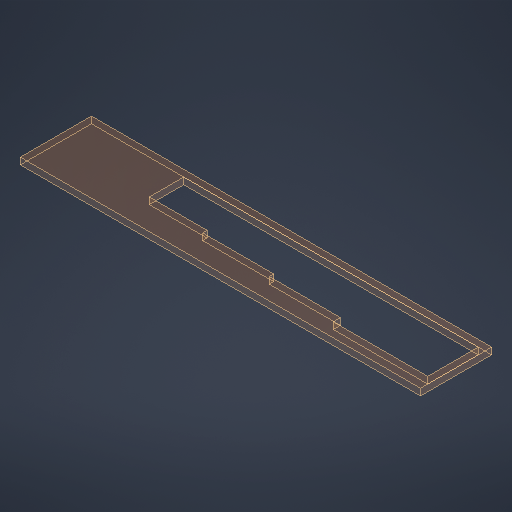
# Autodesk Inventor part: sledPlate
Saved by Autodesk Inventor 2026.1 (Build 301233020, 233B)
## iProperties
Created: 2025-11-01
Part Number: sledPlate
Material: Polycarbonate, Smoke
Document SubType Name: Modeling
Designer: Zain
Density: 1.2 g/cm^3
Appearance: Polycarbonate - Smoked
Author: Zain
Autodesk Inventor part; units mm, degrees
ref_plane "YZ Plane" through (0, 0, 0) normal (1, 0, 0) x (0, 1, 0)
ref_plane "XZ Plane" through (0, 0, 0) normal (0, 1, 0) x (-1, 0, 0)
ref_plane "XY Plane" through (0, 0, 0) normal (0, 0, 1) x (1, 0, 0)
sketch "Sketch1" plane through (0, 0, 0) normal (0, 1, 0) x (-1, 0, 0)
  line L0 (0, 0) -> (180, 0)
  line L1 (180, 0) -> (180, -32)
  line L2 (180, -32) -> (0, -32)
  line L3 (0, -32) -> (0, 0)
  line L4 (0, -32) -> (180, -32)
  line L5 (180, -32) -> (180, -29)
  line L6 (180, -29) -> (0, -29)
  line L7 (0, -29) -> (0, -32)
  line L8 (0, -32) -> (3, -32)
  line L9 (3, -32) -> (3, 0)
  line L10 (3, 0) -> (0, 0)
  line L11 (0, 0) -> (0, -32)
  line L12 (135.5, -29) -> (109.5, -29)
  line L13 (109.5, -29) -> (109.5, -13.5)
  line L14 (109.5, -13.5) -> (135.5, -13.5)
  line L15 (135.5, -13.5) -> (135.5, -29)
  line L16 (109.5, -29) -> (77.5, -29)
  line L17 (77.5, -29) -> (77.5, -11.5)
  line L18 (77.5, -11.5) -> (109.5, -11.5)
  line L19 (109.5, -11.5) -> (109.5, -29)
  line L20 (77.5, -29) -> (45.5, -29)
  line L21 (45.5, -29) -> (45.5, -9.5)
  line L22 (45.5, -9.5) -> (77.5, -9.5)
  line L23 (77.5, -9.5) -> (77.5, -29)
  line L24 (45.5, -29) -> (3, -29)
  line L25 (3, -29) -> (3, -6.25)
  line L26 (3, -6.25) -> (45.5, -6.25)
  line L27 (45.5, -6.25) -> (45.5, -29)
  point P0 (3, -29)
  point P1 (0, -29)
  dimension "d0" = 180
  dimension "d1" = 32
  dimension "d2" = 3
  dimension "d3" = 3
  dimension "d4" = 26
  dimension "d5" = 42.5
  dimension "d6" = 32
  dimension "d7" = 32
  dimension "d14" = 18.5
  dimension "d16" = 20.5
  dimension "d17" = 22.5
  dimension "d18" = 25.75
  constraints: 56 end point, 14 parallel, 7 horizontal, 7 perpendicular, 4 point on line
  measures "d0" distance of L1.end L2.end
  measures "d1" distance of L2.end L0.start
  measures "d2" distance between parallel lines of L3 L9
  measures "d3" distance between parallel lines of L2 L6
  measures "d4" distance of L13.end L14.end
  measures "d5" distance of L25.end L26.end
  measures "d6" distance of L21.end L22.end
  measures "d7" distance of L17.end L18.end
  measures "d14" distance between parallel lines of L14 L2
  measures "d16" distance between parallel lines of L18 L2
  measures "d17" distance between parallel lines of L2 L22
  measures "d18" distance between parallel lines of L2 L26
extrude "Extrusion1" add sketch "Sketch1" along normal blind 3 contours L0 L9 L6 L3 | L0 L1 L6 L15 L14 L19 L18 L23 L22 L27 L26 L9 | L6 L9 L2 L3 | L6 L1 L2 L9
body "Solid1"
